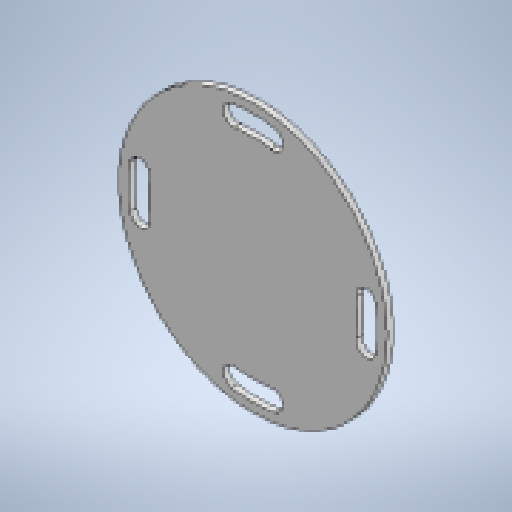
# Autodesk Inventor part: MSC 906 FLANGE FRAME
Saved by Autodesk Inventor 2025 (Build 290162010, 162A)
## iProperties
Created: 2024-07-01
Part Number: MSC 906 FLANGE FRAME
Material: Stainless Steel
Document SubType Name: Sheet Metal
Designer: pokla
Density: 8 g/cm^3
Sheet Metal Rule: AISI304 4mm Die 32
Appearance: Default
Stock Number: МОО 906 фланец рамы
Mass: 715.001 g
Surface Area: 483.276 cm^2
Volume: 89.3752 cm^3
Flat Pattern Width: 17.5 cm
Flat Pattern Length: 17.5 cm
Flat Pattern Area: 306.25 cm^2
Sheet Metal Width: 175,000 mm
Sheet Metal Length: 175,000 mm
Sheet Metal Area: 30625,000 mm^2
Author: pokla
Autodesk Inventor part; units mm, degrees
ref_plane "YZ Plane" through (0, 0, 0) normal (1, 0, 0) x (0, 1, 0)
ref_plane "XZ Plane" through (0, 0, 0) normal (0, 1, 0) x (-1, 0, 0)
ref_plane "XY Plane" through (0, 0, 0) normal (0, 0, 1) x (1, 0, 0)
sketch "Sketch1" plane through (0, 0, 0) normal (0, 1, 0) x (-1, 0, 0)
  circle A0 centre (0, 0) radius 87.5
  dimension "d0" = 175
  measures "d0" diameter of A0
extrude "Plate1" add sketch "Sketch1" along normal blind 4
sketch "Sketch2" plane through (0, 4, 0) normal (0, 1, 0) x (1, 0, 0)
  circle A0 centre (0, 0) radius 87.5 projected
  arc A1 (73.3682, -12.9368) -> (73.3682, 12.9368) centre (0, 0) ccw construction
  arc A2 (79.7694, -14.0655) -> (79.7694, 14.0655) centre (0, 0) ccw
  arc A3 (66.9669, -11.8081) -> (66.9669, 11.8081) centre (0, 0) ccw
  arc A4 (66.9669, -11.8081) -> (79.7694, -14.0655) centre (73.3682, -12.9368) ccw
  arc A5 (79.7694, 14.0655) -> (66.9669, 11.8081) centre (73.3682, 12.9368) ccw
  point P0 (74.5, 0)
  dimension "d19" = 13
  dimension "d20" = 20
  dimension "d21" = 74.5
  constraints: 11 point on circle, 5 centre point, 4 tangent, 2 coincident, 1 horizontal alignment
  measures "d19" diameter of A4
  measures "d21" radius of A1
extrude "Extrusion1" cut sketch "Sketch2" against normal through all contours A4 A3 A5 A2
pattern_circular "Circular Pattern1" count 4 over 360 about axis through (0, -10, 0) along (0, 1, 0) of "Extrusion1"
sketch "Sketch3" plane through (0, 4, 0) normal (0, 1, 0) x (1, 0, 0)
  line L0 (40.5, 40.5) -> (-40.5, 40.5)
  line L1 (-40.5, 40.5) -> (-40.5, -40.5)
  line L2 (-40.5, -40.5) -> (40.5, -40.5)
  line L3 (40.5, -40.5) -> (40.5, 40.5)
  line L4 (40.5, 40.5) -> (-40.5, -40.5) construction
  line L5 (-40.5, 40.5) -> (40.5, -40.5) construction
  point P0 (0, 0)
  dimension "d22" = 81
  constraints: 12 end point, 2 midpoint, 2 parallel, 2 perpendicular, 1 horizontal
  measures "d22" distance of L2.end L1.end
mark "Mark1"
equation "\"d1\" = Thickness"
equation "\"BendReliefWidth\" = Thickness"
equation "\"BendReliefDepth\" = 0.5 * Thickness"
equation "\"CornerReliefSize\" = 4 * Thickness"
equation "\"MinimumRemnant\" = 2 * Thickness"
equation "\"TransitionRadius\" = BendRadius"
equation "\"JacobiRadiusSize\" = BendRadius"
equation "\"GapSize\" = Thickness"
equation "\"Thickness\" = 4"
equation "\"BendRadius\" = 6"
body "Solid1"
